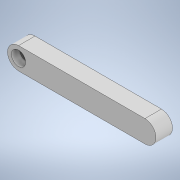
# Autodesk Inventor part: foot
Saved by Autodesk Inventor 2022 (Build 260153000, 153)
## iProperties
Created: 2021-01-08
Part Number: foot
Material: Generic
Document SubType Name: Modeling
Designer: papa
Density: 1 g/cm^3
Appearance: Default
Author: papa
Autodesk Inventor part; units mm, degrees
ref_plane "YZ Plane" through (0, 0, 0) normal (1, 0, 0) x (0, 1, 0)
ref_plane "XZ Plane" through (0, 0, 0) normal (0, 1, 0) x (-1, 0, 0)
ref_plane "XY Plane" through (0, 0, 0) normal (0, 0, 1) x (1, 0, 0)
sketch "Sketch1" plane through (0, 0, 0) normal (0, 0, 1) x (1, 0, 0)
  line L0 (0, 0) -> (46, 0) construction
  line L1 (0, -4) -> (46, -4)
  line L2 (46, 4) -> (0, 4)
  arc A0 (0, 4) -> (0, -4) centre (0, 0) ccw
  arc A1 (46, -4) -> (46, 4) centre (46, 0) ccw
  circle A2 centre (0, 0) radius 1.5
  point P0 (23, 0)
  dimension "d0" = 46
  dimension "d1" = 3
  constraints: 8 end point, 4 point on circle, 4 tangent, 3 centre point, 1 coincident, 1 horizontal, 1 midpoint, 1 parallel
  measures "d0" distance of L0.start L0.end
  measures "d1" diameter of A2
extrude "Extrusion1" add sketch "Sketch1" along normal blind 6
sketch "Sketch2" plane through (0, 0, 6) normal (0, 0, 1) x (1, 0, 0)
  circle A0 centre (0, 0) radius 2.6
  dimension "d4" = 5.2
  constraints: 1 centre point, 1 coincident
  measures "d4" diameter of A0
extrude "Extrusion2" cut sketch "Sketch2" against normal blind 3
body "Solid1"
